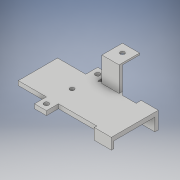
# Autodesk Inventor part: New shifted poe ethernet splitter holder
Saved by Autodesk Inventor 2018 (Build 220112000, 112)
## iProperties
Created: 2019-11-08
Part Number: New shifted poe ethernet splitter holder
Material: Generic
Document SubType Name: Modeling
Designer: Jacob
Density: 1 g/cm^3
Appearance: Default
Author: Jacob
Autodesk Inventor part; units mm, degrees
ref_plane "YZ Plane" through (0, 0, 0) normal (1, 0, 0) x (0, 1, 0)
ref_plane "XZ Plane" through (0, 0, 0) normal (0, 1, 0) x (-1, 0, 0)
ref_plane "XY Plane" through (0, 0, 0) normal (0, 0, 1) x (1, 0, 0)
sketch "Sketch1" plane through (0, 0, 0) normal (0, 1, 0) x (-1, 0, 0)
  line L0 (5, -5) -> (-5, -5)
  line L1 (-5, -5) -> (-5, 5)
  line L2 (-5, 5) -> (5, 5)
  line L3 (5, 5) -> (5, -5)
  line L4 (5, -5) -> (-5, 5) construction
  line L5 (-5, -5) -> (5, 5) construction
  circle A0 centre (0, 0) radius 1.5
  dimension "d0" = 10
  dimension "d1" = 10
  dimension "d2" = 3
  constraints: 12 end point, 2 midpoint, 2 parallel, 1 centre point, 1 coincident, 1 horizontal, 1 perpendicular
  measures "d0" distance of L0.start L0.end
  measures "d1" distance of L0.end L1.end
  measures "d2" diameter of A0
extrude "Extrusion1" add sketch "Sketch1" along normal blind 1
sketch "Sketch2" plane through (0, 1, 0) normal (0, 1, 0) x (1, 0, 0)
  line L0 (5, 5) -> (-5, 5) projected
  line L1 (-5, 5) -> (5, 5)
  line L2 (5, 5) -> (5, 6.5)
  line L3 (5, 6.5) -> (-5, 6.5)
  line L4 (-5, 6.5) -> (-5, 5)
  point P0 (0, 0)
  dimension "d5" = 1.5
  constraints: 8 end point, 2 parallel, 1 horizontal, 1 perpendicular
  measures "d5" distance of L1.end L2.end
extrude "Extrusion2" add sketch "Sketch2" against normal blind 1
sketch "Sketch3" plane through (0, 1, 0) normal (0, 1, 0) x (1, 0, 0)
  line L0 (-5, 6.5) -> (-5, -5) projected
  line L1 (5, -5) -> (5, 6.5) projected
  line L2 (-5, 6.5) -> (5, 6.5)
  line L3 (5, 6.5) -> (5, 5)
  line L4 (5, 5) -> (-5, 5)
  line L5 (-5, 5) -> (-5, 6.5)
  point P0 (0, 0)
  dimension "d8" = 1.5
  constraints: 8 end point, 2 parallel, 1 horizontal, 1 perpendicular, 1 point on line
  measures "d8" distance between parallel lines of L2 L4
extrude "Extrusion3" add sketch "Sketch3" along normal blind 17
sketch "Sketch4" plane through (0, 18, 0) normal (0, 1, 0) x (1, 0, 0)
  line L0 (-5, 5) -> (5, 5) projected
  line L1 (5, 6.5) -> (-5, 6.5) projected
  line L2 (-5, 6.5) -> (-5, 5) projected
  line L3 (5, 5) -> (5, 6.5) projected
  point P0 (0, 0)
extrude "Extrusion4" add sketch "Sketch4" along normal blind 1.5
sketch "Sketch5" plane through (5, 0, -6.5) normal (0, 0, -1) x (-1, 0, 0)
  line L0 (0, 19.5) -> (10, 19.5) projected
  line L1 (0, 19.5) -> (56, 19.5)
  line L2 (56, 19.5) -> (56, 18)
  line L3 (56, 18) -> (0, 18)
  line L4 (0, 18) -> (0, 19.5)
  line L5 (0, 19.5) -> (56, 18) construction
  line L6 (56, 19.5) -> (0, 18) construction
  line L7 (0, 0) -> (0, 19.5) projected
  point P0 (5, 0)
  point P1 (28, 18.75)
  dimension "d13" = 0
  dimension "d14" = 1.5
  dimension "d15" = 56
  dimension "d42" = 0
  constraints: 12 end point, 2 midpoint, 2 parallel, 1 horizontal, 1 perpendicular
  measures "d13" distance between parallel lines of L0 L1
  measures "d14" distance of L3.end L1.start
  measures "d15" distance of L2.end L3.end
  measures "d42" distance between parallel lines of L7 L4
extrude "Extrusion5" add sketch "Sketch5" along normal blind 23
sketch "Sketch11" plane through (0, 19.5, 0) normal (0, 1, 0) x (1, 0, 0)
  line L0 (-51, 6.5) -> (-51, 29.5) projected
  line L1 (-51, 18) -> (5, 18) construction
  line L2 (5, 6.5) -> (5, 29.5) projected
  line L3 (-5, 6.5) -> (-51, 6.5) projected
  line L4 (-5, 5) -> (5, 5) projected
  line L5 (-5, 6.5) -> (-5, 5) projected
  line L6 (5, 5) -> (5, 29.5) projected
  line L7 (-51, 29.5) -> (5, 29.5) projected
  circle A0 centre (-31, 18) radius 1.25
  point P0 (0, 0)
  dimension "d45" = 2.5
  dimension "d46" = 20
  constraints: 2 end point, 2 midpoint, 1 centre point, 1 point on line
  measures "d45" diameter of A0
  measures "d46" distance from line of L0 A0.centre
extrude "Extrusion10" add sketch "Sketch11" along normal blind 1
sketch "Sketch12" plane through (0, 20.5, 0) normal (0, 1, 0) x (1, 0, 0)
  line L0 (5, 29.5) -> (-51, 29.5) projected
  line L1 (-51, 6.5) -> (-5, 6.5) projected
  line L2 (5, 29.5) -> (-51, 29.5) projected
  line L3 (-31, 29.5) -> (-31, 6.5) construction
  line L4 (-51, 6.5) -> (-5, 6.5) projected
  line L5 (-51, 29.5) -> (-51, 6.5) projected
  line L6 (-31, 29.5) -> (-31, 36.5) construction
  line L7 (-31, 6.5) -> (-31, -12.5125) construction
  line L8 (-34.5, 6.5) -> (-27.5, 6.5)
  line L9 (-27.5, 6.5) -> (-27.5, -0.5)
  line L10 (-27.5, -0.5) -> (-34.5, -0.5)
  line L11 (-34.5, -0.5) -> (-34.5, 6.5)
  line L12 (-34.5, 6.5) -> (-27.5, -0.5) construction
  line L13 (-27.5, 6.5) -> (-34.5, -0.5) construction
  line L14 (-34.5, 36.5) -> (-27.5, 36.5)
  line L15 (-27.5, 36.5) -> (-27.5, 29.5)
  line L16 (-27.5, 29.5) -> (-34.5, 29.5)
  line L17 (-34.5, 29.5) -> (-34.5, 36.5)
  line L18 (-34.5, 36.5) -> (-27.5, 29.5) construction
  line L19 (-27.5, 36.5) -> (-34.5, 29.5) construction
  circle A0 centre (-31, 33) radius 1.375
  circle A1 centre (-31, 3) radius 1.375
  point P0 (0, 0)
  dimension "d49" = 20
  dimension "d50" = 0
  dimension "d51" = 0
  dimension "d52" = 7
  dimension "d53" = 7
  dimension "d54" = 7
  dimension "d55" = 7
  dimension "d56" = 2.75
  dimension "d57" = 2.75
  constraints: 30 end point, 5 midpoint, 4 parallel, 3 perpendicular, 3 point on line, 2 centre point, 2 coincident, 2 horizontal, 2 vertical
  measures "d49" distance between parallel lines of L3 L5
  measures "d50" distance between parallel lines of L0 L16
  measures "d51" distance between parallel lines of L4 L8
  measures "d52" distance of L14.start L14.end
  measures "d53" distance of L14.end L15.end
  measures "d54" distance of L8.end L9.end
  measures "d55" distance of L9.end L10.end
  measures "d56" diameter of A0
  measures "d57" diameter of A1
extrude "Extrusion11" add sketch "Sketch12" against normal blind 2.5
sketch "Sketch13" plane through (0, 20.5, 0) normal (0, 1, 0) x (1, 0, 0)
  line L0 (-5, -5) -> (5, -5) projected
  line L1 (0, -5) -> (0, 55.8015) construction
  line L2 (-5, 29.5) -> (5, 29.5)
  line L3 (5, 29.5) -> (5, 32.5)
  line L4 (5, 32.5) -> (-5, 32.5)
  line L5 (-5, 32.5) -> (-5, 29.5)
  line L6 (-5, 29.5) -> (5, 32.5) construction
  line L7 (5, 29.5) -> (-5, 32.5) construction
  line L8 (5, 29.5) -> (-27.5, 29.5) projected
  point P0 (0, 0)
  point P1 (0, 31)
  dimension "d60" = 0
  dimension "d61" = 3
  dimension "d62" = 10
  constraints: 14 end point, 3 midpoint, 2 parallel, 1 horizontal, 1 perpendicular, 1 point on line, 1 vertical
  measures "d60" distance between parallel lines of L8 L2
  measures "d61" distance of L4.end L2.start
  measures "d62" distance of L3.end L4.end
extrude "Extrusion12" add sketch "Sketch13" against normal blind 10
sketch "Sketch14" plane through (-5, 18, -29.5) normal (0, 0, 1) x (1, 0, 0)
  line L0 (0, 0) -> (-46, 0) projected
  line L1 (10, -7.5) -> (0, -7.5) projected
  line L2 (0, 0) -> (10, 0)
  line L3 (10, 0) -> (10, -7.5)
  line L4 (10, -7.5) -> (0, -7.5)
  line L5 (0, -7.5) -> (0, 0)
  point P0 (5, -18)
  constraints: 8 end point, 2 parallel, 1 horizontal, 1 perpendicular
extrude "Extrusion13" cut sketch "Sketch14" against normal blind 1
sketch "Sketch15" plane through (-5, 1, -5) normal (0, 0, 1) x (1, 0, 0)
  line L0 (-46, 17) -> (0, 17) projected
  line L1 (0, 0) -> (0, 19.5) projected
  line L2 (10, 0) -> (10, 19.5) projected
  line L3 (10, -1) -> (0, -1) projected
  line L4 (0, -1) -> (0, 17) projected
  line L5 (10, -1) -> (10, 17) projected
  line L6 (0, 13) -> (10, 13)
  line L7 (10, 13) -> (10, -1)
  line L8 (10, -1) -> (0, -1)
  line L9 (0, -1) -> (0, 13)
  point P0 (5, -1)
  dimension "d67" = 4
  dimension "d68" = 0
  constraints: 8 end point, 2 parallel, 2 point on line, 1 horizontal, 1 perpendicular
  measures "d67" distance between parallel lines of L0 L6
  measures "d68" distance between parallel lines of L3 L8
extrude "Extrusion14" cut sketch "Sketch15" along normal mid plane 20
sketch "Sketch19" plane through (0, 20.5, 0) normal (0, 1, 0) x (1, 0, 0)
  circle A0 centre (-31, 18) radius 1.25 projected
  point P0 (0, 0)
extrude "Extrusion18" cut sketch "Sketch19" along normal mid plane 30
sketch "Sketch24" plane through (0, 20.5, 0) normal (0, 1, 0) x (1, 0, 0)
  line L0 (-5, 29.5) -> (-27.5, 29.5) projected
  line L1 (-15, 29.5) -> (-25, 29.5)
  line L2 (-25, 29.5) -> (-25, 31.5)
  line L3 (-25, 31.5) -> (-15, 31.5)
  line L4 (-15, 31.5) -> (-15, 29.5)
  line L5 (5, 5) -> (5, 32.5) projected
  point P0 (0, 0)
  dimension "d95" = 20
  dimension "d96" = 10
  dimension "d97" = 2
  constraints: 8 end point, 2 parallel, 1 horizontal, 1 perpendicular, 1 point on line
  measures "d95" distance between parallel lines of L4 L5
  measures "d96" distance between parallel lines of L4 L2
  measures "d97" distance of L3.end L1.start
extrude "Extrusion23" add sketch "Sketch24" along normal blind 14.5
sketch "Sketch25" plane through (0, 20.5, 0) normal (0, -1, 0) x (1, 0, 0)
  line L0 (-25, -29.5) -> (-25, -31.5) projected
  line L1 (-15, -29.5) -> (-25, -29.5) projected
  line L2 (-25, -29.5) -> (-25, -31.5) projected
  line L3 (-25, -31.5) -> (-15, -31.5) projected
  line L4 (-15, -31.5) -> (-15, -29.5) projected
  point P0 (0, 0)
extrude "Extrusion24" add sketch "Sketch25" along normal blind 2.5
sketch "Sketch26" plane through (-15, 35, -31.5) normal (0, 0, -1) x (-1, 0, 0)
  line L0 (0, 0) -> (10, 0) projected
  line L1 (0, 0) -> (0, -17) projected
  line L2 (10, 0) -> (0, 0)
  line L3 (0, 0) -> (0, -1)
  line L4 (0, -1) -> (10, -1)
  line L5 (10, -1) -> (10, 0)
  point P0 (-15, -35)
  dimension "d102" = 1
  constraints: 8 end point, 2 parallel, 1 horizontal, 1 perpendicular, 1 point on line
  measures "d102" distance between parallel lines of L4 L0
extrude "Extrusion25" add sketch "Sketch26" along normal blind 10
sketch "Sketch27" plane through (-25, 34, -31.5) normal (0, -1, 0) x (1, 0, 0)
  line L0 (0, 0) -> (0, -10) projected
  line L1 (0, -5) -> (10, -5) construction
  line L2 (10, 0) -> (10, -10) projected
  line L3 (0, 0) -> (10, 0) projected
  line L4 (0, 0) -> (10, 0) projected
  line L5 (0, 0) -> (0, -10) projected
  line L6 (10, -10) -> (0, -10) projected
  line L7 (10, 0) -> (10, -10) projected
  line L8 (5, 0) -> (5, -10) construction
  circle A0 centre (5, -5) radius 1.25
  point P0 (25, 31.5)
  dimension "d105" = 2.5
  constraints: 5 midpoint, 4 end point, 1 centre point
  measures "d105" diameter of A0
extrude "Extrusion26" cut sketch "Sketch27" against normal blind 10 contours A0
chamfer "Chamfer1" distance 2 angle 45 2 edges at (-15, 19.25, -29.5) (-25, 19.25, -29.5)
body "Solid1"
